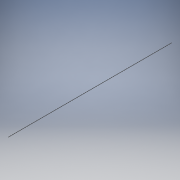
# Autodesk Inventor part: 2829-CL-5
Saved by Autodesk Inventor 2019 (Build 230136000, 136)
## iProperties
Category: PARTsolutions
Company: 8020
Created: 2019-03-04
Part Number: 2829-CL-5
Material: Generic
Catalog Web Link: www.cadenas.de
Description: 2829-Rubber Door Seal
Vendor: 8020
Document SubType Name: Modeling
Designer: psadmin
Manufacturer: 8020
Mass: 0.212265 g
Surface Area: 84.8839 cm^2
Volume: 0.212265 cm^3
Density: 1 g/cm^3
Appearance: PSOLRGB-0-0-0
PSOL_IDENT_0: {$CADENAS_DATA\23d-libs\8020\inch\panels_and_doors\2829.prj},158 {VTYP=3D},{NB=2829-CL-5},{LINA=2829
PSOL_IDENT_1: -5},{NN=2829},{DATE=04.12.2018 10:30:19},{GEOMDATE=02.03.2018 10:35:21},{VERSION=},{LINEID=10},{WBVA
PSOL_IDENT_2: R=LS,L},{WBNUMERIC=L}  {NB=2829-CL-5},{LINA=2829-5},{KT=DUMMY},{PN=2829},{SERIES=15 / 40},{LS=CL},{L=
PSOL_IDENT_3: 5.000},{A=0.17000},{B=0.32200},{C=0.75000},{D=0.74200},{E=0.32000},{F=0.53000},{LENGTH=per foot},{WE
PSOL_IDENT_4: IGHT=0.090 lb / ft},{LALG=[1:100/1.000]}
NN: 2829
NT: Rubber Door Seal
NB: 2829-CL-5
NBSYN: $PN.-$LS.-$L.
LINA: 2829-5
PN: 2829
SERIES: 15 / 40
LS: Custom length
L: 5
A: 0.17
B: 0.322
C: 0.75
D: 0.742
E: 0.32
F: 0.53
LENGTH: per foot
WEIGHT: 0.090 lb / ft
SUPPLIER: 8020
ARTICLENO: 2829-CL-5
BOMINFO: 2829-5
CREATOR: CADENAS GmbH
Title: 2829-5
Author: Cadenas PARTsolutions
Comments: Rubber Door Seal
Autodesk Inventor part; units mm, degrees
ref_plane "YZ Plane" through (0, 0, 0) normal (1, 0, 0) x (0, 1, 0)
ref_plane "XZ Plane" through (0, 0, 0) normal (0, 1, 0) x (-1, 0, 0)
ref_plane "XY Plane" through (0, 0, 0) normal (0, 0, 1) x (1, 0, 0)
sketch "Sketch_1" plane through (0, 0, 0) normal (0, 0, 1) x (1, 0, 0)
  arc A0 (-0.2225, 0.606) -> (-0.375, 0.42) centre (-0.1915, 0.425) ccw
  line L0 (-0.375, 0.42) -> (-0.195, 0.42)
  arc A1 (-0.16, 0.385) -> (-0.195, 0.42) centre (-0.195, 0.385) ccw
  line L1 (-0.16, 0.385) -> (-0.16, 0.285)
  arc A2 (-0.195, 0.25) -> (-0.16, 0.285) centre (-0.195, 0.285) ccw
  line L2 (-0.195, 0.25) -> (-0.265, 0.25)
  line L3 (-0.265, 0.25) -> (-0.265, 0.1899)
  arc A3 (-0.265, 0.1899) -> (-0.2521, 0.1563) centre (-0.215, 0.1899) ccw
  line L4 (-0.2521, 0.1563) -> (-0.1254, 0.0164)
  arc A4 (-0.1254, 0.0164) -> (-0.0884, 0) centre (-0.0884, 0.05) ccw
  line L5 (-0.0884, 0) -> (0.0884, 0)
  arc A5 (0.0884, 0) -> (0.1254, 0.0164) centre (0.0884, 0.05) ccw
  line L6 (0.1254, 0.0164) -> (0.2521, 0.1563)
  arc A6 (0.2521, 0.1563) -> (0.265, 0.1899) centre (0.215, 0.1899) ccw
  line L7 (0.265, 0.1899) -> (0.265, 0.25)
  line L8 (0.265, 0.25) -> (0.195, 0.25)
  arc A7 (0.16, 0.285) -> (0.195, 0.25) centre (0.195, 0.285) ccw
  line L9 (0.16, 0.285) -> (0.16, 0.385)
  arc A8 (0.195, 0.42) -> (0.16, 0.385) centre (0.195, 0.385) ccw
  line L10 (0.195, 0.42) -> (0.375, 0.42)
  arc A9 (0.375, 0.42) -> (0.2225, 0.606) centre (0.1915, 0.425) ccw
  arc A10 (0.2225, 0.606) -> (-0.2225, 0.606) centre (0, 0.492) ccw
  line L11 (-0.11, 0.42) -> (-0.11, 0.05)
  line L12 (-0.11, 0.05) -> (0.11, 0.05)
  line L13 (0.11, 0.05) -> (0.11, 0.42)
  line L14 (0.11, 0.42) -> (-0.11, 0.42)
  line L15 (-0.337, 0.455) -> (0.337, 0.455)
  arc A11 (0.337, 0.455) -> (0.2221, 0.5704) centre (0.1915, 0.425) ccw
  arc A12 (0.1885, 0.5954) -> (0.2221, 0.5704) centre (0.2324, 0.6194) ccw
  arc A13 (0.1885, 0.5954) -> (-0.1885, 0.5954) centre (0, 0.492) ccw
  arc A14 (-0.2221, 0.5704) -> (-0.1885, 0.5954) centre (-0.2324, 0.6194) ccw
  arc A15 (-0.2221, 0.5704) -> (-0.337, 0.455) centre (-0.1915, 0.425) ccw
  constraints: 32 end point, 32 point on circle, 16 centre point
extrude "Extrusion1" add sketch "Sketch_1" along normal mid plane 762
body "Solid1"
